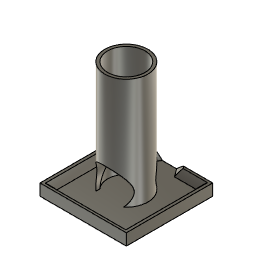
toothbrush v2 (Autodesk Fusion 360 design; units mm, degrees)
Autodesk Fusion 360 part; units mm, degrees
note: some values were not read from the file. Chosen so that the rebuilt part matches the saved one: which face or edge a step refers to; that a step has no effect.
cylinder "円柱プリミティブ2" add diameter 15 height 40 placed x (1, 0, 0) y (0, 1, 0) z (0, 0, 1) at (0, 0, 0) makes body 1
hole "穴1" at (0, 0, 40) direction (0, 0, -1) diameter 13 depth 50 tip angle 118 bodies 1
box "直方体プリミティブ1" add length 30 width 30 height 2 placed x (0, 1, 0) y (-1, 0, 0) z (0, 0, 1) at (30, 0, 0) separate body makes body 2
move_face "面を移動1" [no effect]
move_face "面を移動2" by (-10, 0, 0) 1 faces at (20, 0, 0.6667) on bodies 2
move_face "面を移動3" [no effect]
move_body "移動1" bodies 2 to x (1, 0, 0) y (0, 1, 0) z (0, 0, 1) at (-15, -15, 0)
hole "穴2" at (0, -7.5, 5.8844) direction (0, 1, 0) diameter 13 depth 50 tip angle 180 bodies 1
move_body "移動2" bodies 1 to x (1, 0, 0) y (0, 1, 0) z (0, 0, 1) at (0, 0, 0.5)
combine "結合1" operation add target body 1 tool bodies 2
sketch "スケッチ5" plane through (0, 0, 2) normal (0, 0, 1) x (-1, 0, 0)
  line L0 (-15, -15) -> (15, -15)
  line L1 (15, -15) -> (15, 15)
  line L2 (15, 15) -> (-15, 15)
  line L3 (-15, 15) -> (-15, -15)
  line L4 (-12.01, 12.2) -> (12.01, 12.2)
  line L5 (12.01, 12.2) -> (12.01, -12.2)
  line L6 (12.01, -12.2) -> (-12.01, -12.2)
  line L7 (-12.01, -12.2) -> (-12.01, 12.2)
  line L8 (-12.01, 12.2) -> (12.01, -12.2) construction
  line L9 (12.01, 12.2) -> (-12.01, -12.2) construction
  line L10 (4.7986, -5.7639) -> (4.7986, -4.3844)
  line L11 (4.7986, 4.3844) -> (4.7986, 5.7639)
  line L12 (-15, 15) -> (15, 15)
  line L13 (15, 15) -> (15, -15)
  line L14 (15, -15) -> (-15, -15)
  line L15 (-15, -15) -> (-15, 15)
  line L16 (-15, 15) -> (15, -15) construction
  line L17 (15, 15) -> (-15, -15) construction
  line L18 (0, -12.2) -> (0, -15) construction
  line L19 (4.5, -12.2) -> (2.5, -15)
  line L20 (-4.5, -12.2) -> (-2.5, -15)
  arc A0 (4.7986, -5.7639) -> (4.7986, 5.7639) centre (0, 0) ccw
  arc A1 (4.7986, -4.3844) -> (4.7986, 4.3844) centre (0, 0) ccw
  line L21 (-4.7986, 5.7639) -> (-4.7986, 4.3844)
  arc A2 (-4.7986, 4.3844) -> (-4.7986, -4.3844) centre (0, 0) ccw
  line L22 (-4.7986, -4.3844) -> (-4.7986, -5.7639)
  arc A3 (-4.7986, 5.7639) -> (-4.7986, -5.7639) centre (0, 0) ccw
  constraint horizontal L4
  constraint perpendicular L4 L5
  constraint parallel L4 L6
  constraint parallel L5 L7
  constraint coincident L8 A0.centre
  constraint coincident L9 A0.centre
  constraint coincident A0.centre A1.centre
  constraint horizontal L12
  constraint perpendicular L12 L13
  constraint parallel L12 L14
  constraint parallel L13 L15
  constraint coincident L16 A0.centre
  constraint coincident L17 A0.centre
  constraint coincident L2.end L3.start
  constraint midpoint L6 L18.start
  constraint midpoint L14 L18.end
  constraint coincident L6 L19.start
  constraint coincident L14 L19.end
  constraint symmetric L18 L19.start L20.start
  constraint symmetric L18 L19.end L20.end
extrude "押し出し1" add sketch "スケッチ5" along normal blind 1 contours L0 L1 L2 L3 L4 L5 L6 L7 L12 L13 L14 L15 L19 L20 bodies 1
extrude "押し出し2" add 1 faces at (-14.0033, -4.0667, 3) along direction (0, 0, 1) blind 1 on bodies 1 bodies 1
fillet "フィレット1" radius 2 tangency weight 0.1 7 edges at (-12.01, 0, 4) (0, -12.2, 4) (12.01, 0, 4) (8.255, 12.2, 4) (3.5, 13.6, 4) (-3.5, 13.6, 4) (-8.255, 12.2, 4) on bodies 1
